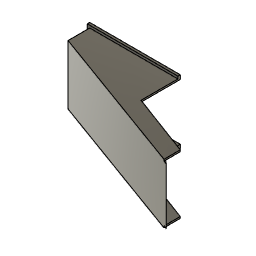
Food_Chute v4 (Autodesk Fusion 360 design; units mm, degrees)
Autodesk Fusion 360 part; units mm, degrees
sketch "Sketch1" plane through (0, 0, 0) normal (0, 0, 1) x (1, 0, 0)
  line L0 (0, 0) -> (0, 30)
  line L1 (0, 0) -> (192.637, -70.1141)
  line L2 (0, 0) -> (200, 0) construction
  line L3 (192.637, -70.1141) -> (188.0053, -66.3)
  line L4 (192.637, -70.1141) -> (203.3355, -70.1141) construction
  line L5 (188.0053, -66.3) -> (2, 1.4004)
  line L6 (0, 30) -> (2, 30)
  line L7 (2, 30) -> (2, 1.4004)
  dimension "d2" = 30
  dimension "d3" = 20
  dimension "d4" = 205
  dimension "d6" = 6
  dimension "d10" = 2
  dimension "d13" = 140.529
  constraint coincident L0.start L1.start
  constraint vertical L0
  constraint horizontal L2
  constraint horizontal L4
  constraint perpendicular L0 L6
  constraint perpendicular L2 L7
  constraint parallel L1 L5
  measures "d2" distance of L0.start L0.end
  measures "d3" angle of L1 L2
  measures "d4" distance of L0.start L1.end
  measures "d6" distance of L1.end L3.end
  measures "d10" distance of L0.end L6.end
  measures "d13" angle of L3 L4
extrude "Extrude1" add sketch "Sketch1" along normal blind 70 makes body 1
sketch "Sketch2" plane through (0, 0, 0) normal (0, 0, 1) x (1, 0, 0)
  line L0 (2, 1.4004) -> (2, 30)
  line L1 (0, 30) -> (110, 30)
  line L2 (110, 30) -> (110, -19.0179)
  line L3 (110, -19.0179) -> (188.0053, -48.1069)
  line L4 (188.0053, -66.3) -> (188.0053, -48.1069)
  line L5 (2, 30) -> (0, 30)
  line L6 (0, 30) -> (0, 0)
  line L7 (0, 30) -> (0, 29)
  line L8 (0, 0) -> (192.637, -70.1141)
  line L9 (0, 0) -> (192.7051, -70.1389)
  line L10 (188.0053, -66.3) -> (188.0053, -68.4283)
  point P0 (2, 30)
  point P1 (188.0053, -66.3)
  point P2 (0, 30)
  dimension "d16" = 110
  constraint perpendicular L0 L1
  constraint perpendicular L1 L2
  constraint coincident P1 L4.start
  constraint coincident L3 L4.end
  constraint vertical L4
  constraint coincident P2 L1.start
  constraint coincident L6 L7.end
  constraint perpendicular L5 L7
  constraint coincident L6.end L8.start
  constraint coincident L8 L9.end
  constraint vertical L10
  constraint coincident L9 L10.end
  measures "d16" distance of P2 L1.end
extrude "Extrude2" add sketch "Sketch2" against normal blind 2 bodies 1
ref_plane "WorkPlane1" through (0, 0, 35) normal (0, 0, 1) x (1, 0, 0)
mirror "Mirror1" about plane through (0, 0, 35) normal (0, 0, 1) of bodies 1 makes body 2
sketch "Sketch3" plane through (0, 0, 72) normal (0, 0, 1) x (-1, 0, 0)
  line L0 (-110, -30) -> (0, -30)
  line L1 (0, -30) -> (0, 0)
  line L2 (0, 0) -> (-188.0053, 68.4283)
  line L3 (-188.0053, 68.4283) -> (-188.0053, 48.1069)
  line L4 (-188.0053, 48.1069) -> (-110, 19.0179)
  line L5 (-110, 19.0179) -> (-110, -30)
  line L6 (0, -30) -> (-110, -30)
  line L7 (-110, -30) -> (-110, -27)
  line L8 (-110, -27) -> (0, -27)
  line L9 (0, -27) -> (0, -30)
  dimension "d22" = 3
  constraint horizontal L6
  constraint vertical L7
  constraint horizontal L8
  constraint vertical L9
  constraint coincident L5 L7.end
  constraint coincident L0.end L1.start
  measures "d22" distance of L0.start L7.end
extrude "Extrude3" add sketch "Sketch3" along normal blind 3 contours L0 L1 L5 L6 L7 L8 L9 bodies 2
sketch "Sketch4" plane through (0, 0, -2) normal (0, 0, -1) x (1, 0, 0)
  line L0 (0, -30) -> (110, -30)
  line L1 (110, -30) -> (110, 19.0179)
  line L2 (110, 19.0179) -> (188.0053, 48.1069)
  line L3 (188.0053, 48.1069) -> (188.0053, 68.4283)
  line L4 (188.0053, 68.4283) -> (0, 0)
  line L5 (0, 0) -> (0, -30)
  line L6 (110, -30) -> (0, -30)
  line L7 (0, -30) -> (0, -27)
  line L8 (0, -27) -> (110, -27)
  line L9 (110, -27) -> (110, -30)
  dimension "d25" = 3
  constraint horizontal L6
  constraint vertical L7
  constraint horizontal L8
  constraint vertical L9
  constraint coincident L5 L7.end
  constraint coincident L0.end L1.start
  measures "d25" distance of L0.start L7.end
extrude "Extrude4" add sketch "Sketch4" along normal blind 3 contours L0 L1 L5 L6 L7 L8 L9 bodies 1
sketch "Sketch5" plane through (0, 0, 0) normal (-1, 0, 0) x (0, -1, 0)
  line L0 (0, 0) -> (0, 72)
  line L1 (0, 72) -> (-27, 72)
  line L2 (-27, 72) -> (-27, 75)
  line L3 (-27, 75) -> (-30, 75)
  line L4 (-30, 75) -> (-30, 0)
  line L5 (-30, 0) -> (0, 0)
  line L6 (-30, -5) -> (-27, -5)
  line L7 (-27, -5) -> (-27, 75)
  line L8 (-27, 75) -> (-30, 75)
  line L9 (-30, 75) -> (-30, -5)
  point P0 (-30, -5)
  constraint horizontal L6
  constraint vertical L7
  constraint horizontal L8
  constraint vertical L9
  constraint coincident L2.end L3.start
  constraint coincident P0 L6.start
extrude "Extrude5" add sketch "Sketch5" along normal blind 3 contours L5 L6 L7 L9 | L2 L3 L4 L5 L7 L8 L9 bodies 1 2
